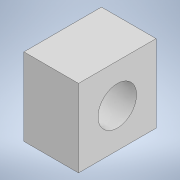
# Autodesk Inventor part: End Piece Corrected 0.02 Inch
Saved by Autodesk Inventor 2022 (Build 260153000, 153)
## iProperties
Created: 2022-01-02
Part Number: End Piece Corrected 0.02 Inch
Material: Generic
Document SubType Name: Modeling
Designer: josephinew
Density: 1 g/cm^3
Appearance: Default
Author: josephinew
Autodesk Inventor part; units mm, degrees
ref_plane "YZ Plane" through (0, 0, 0) normal (1, 0, 0) x (0, 1, 0)
ref_plane "XZ Plane" through (0, 0, 0) normal (0, 1, 0) x (-1, 0, 0)
ref_plane "XY Plane" through (0, 0, 0) normal (0, 0, 1) x (1, 0, 0)
sketch "Sketch1" plane through (0, 0, 0) normal (1, 0, 0) x (0, 1, 0)
  line L0 (18.542, -0.508) -> (0.508, -0.508)
  line L1 (0.508, -0.508) -> (0.508, -18.542)
  line L2 (0.508, -18.542) -> (18.542, -18.542)
  line L3 (18.542, -18.542) -> (18.542, -0.508)
  circle A0 centre (9.525, -9.525) radius 4.4831
  constraints: 8 end point, 2 parallel, 1 centre point, 1 horizontal, 1 perpendicular
extrude "Extrusion1" add sketch "Sketch1" along normal blind 12.7
body "Solid1"
